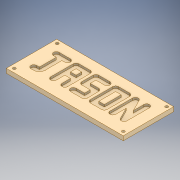
# Autodesk Inventor part: JASON
Saved by Autodesk Inventor 2017 (Build 210142000, 142)
## iProperties
Created: 2016-09-28
Part Number: JASON
Material: Polyethylene, High Density
Document SubType Name: Modeling
Designer: jhaun
Density: 0.952 g/cm^3
Appearance: Smooth - Off-White
Author: jhaun
Autodesk Inventor part; units mm, degrees
ref_plane "YZ Plane" through (0, 0, 0) normal (1, 0, 0) x (0, 1, 0)
ref_plane "XZ Plane" through (0, 0, 0) normal (0, 1, 0) x (-1, 0, 0)
ref_plane "XY Plane" through (0, 0, 0) normal (0, 0, 1) x (1, 0, 0)
sketch "Sketch1" plane through (0, 0, 0) normal (0, 0, 1) x (1, 0, 0)
  arc A0 (0, 6.5) -> (0, -6.5) centre (0, 0) ccw
  line L0 (0, 6.5) -> (26, 6.5)
  line L1 (0, -6.5) -> (6.5, -6.5)
  arc A1 (26, -6.5) -> (26, 6.5) centre (26, 0) ccw
  line L2 (26, -6.5) -> (19.5, -6.5)
  line L3 (6.5, -6.5) -> (6.5, -45.5)
  line L4 (19.5, -6.5) -> (19.5, -45.5)
  line L5 (6.5, -45.5) -> (0, -45.5)
  arc A2 (0, -45.5) -> (0, -58.5) centre (0, -52) ccw
  line L6 (0, -58.5) -> (6.5, -58.5)
  arc A3 (6.5, -58.5) -> (19.5, -45.5) centre (6.5, -45.5) ccw
  line L7 (39, 0) -> (39, -52)
  arc A4 (39, -52) -> (52, -52) centre (45.5, -52) ccw
  line L8 (52, -52) -> (52, -32.5)
  line L9 (52, -32.5) -> (65, -32.5)
  line L10 (52, -6.5) -> (65, -6.5)
  line L11 (65, -6.5) -> (65, -19.5)
  line L12 (65, -19.5) -> (52, -19.5)
  line L13 (52, -19.5) -> (52, -6.5)
  line L14 (45.5, 6.5) -> (71.5, 6.5)
  line L15 (78, 0) -> (78, -52)
  line L16 (65, -32.5) -> (65, -52)
  arc A5 (65, -52) -> (78, -52) centre (71.5, -52) ccw
  arc A6 (45.5, 6.5) -> (39, 0) centre (45.5, 0) ccw
  arc A7 (78, 0) -> (71.5, 6.5) centre (71.5, 0) ccw
  line L17 (84.5, 0) -> (84.5, -26)
  arc A8 (91, 6.5) -> (84.5, 0) centre (91, 0) ccw
  line L18 (91, 6.5) -> (117, 6.5)
  line L19 (91, -32.5) -> (110.5, -32.5)
  arc A9 (84.5, -26) -> (91, -32.5) centre (91, -26) ccw
  line L20 (97.5, -6.5) -> (97.5, -19.5)
  line L21 (97.5, -6.5) -> (117, -6.5)
  arc A10 (117, -6.5) -> (117, 6.5) centre (117, 0) ccw
  line L22 (97.5, -19.5) -> (117, -19.5)
  arc A11 (123.5, -26) -> (117, -19.5) centre (117, -26) ccw
  line L23 (123.5, -26) -> (123.5, -52)
  line L24 (110.5, -32.5) -> (110.5, -45.5)
  line L25 (110.5, -45.5) -> (91, -45.5)
  arc A12 (91, -45.5) -> (91, -58.5) centre (91, -52) ccw
  arc A13 (117, -58.5) -> (123.5, -52) centre (117, -52) ccw
  line L26 (91, -58.5) -> (117, -58.5)
  line L27 (130, 0.001) -> (130, -51.999)
  line L28 (143, -6.499) -> (143, -45.499)
  line L29 (143, -6.499) -> (156, -6.499)
  line L30 (156, -6.499) -> (156, -45.499)
  line L31 (156, -45.499) -> (143, -45.499)
  arc A14 (136.5, 6.501) -> (130, 0.001) centre (136.5, 0.001) ccw
  line L32 (136.5, 6.501) -> (162.5, 6.501)
  line L33 (136.5, -58.499) -> (162.5, -58.499)
  arc A15 (162.5, -58.499) -> (169, -51.999) centre (162.5, -51.999) ccw
  line L34 (169, -51.999) -> (169, 0.001)
  arc A16 (169, 0.001) -> (162.5, 6.501) centre (162.5, 0.001) ccw
  line L35 (175.5, 0) -> (175.5, -52)
  arc A17 (175.524, -51.4421) -> (188.5, -52) centre (182, -52) ccw
  line L36 (214.5, -52.025) -> (214.5, 0.086)
  line L37 (188.5, -52) -> (188.5, -27.5463)
  line L38 (188.5, -27.5463) -> (202.1857, -54.9308)
  line L39 (201.5, 0.086) -> (201.5, -24.4787)
  line L40 (201.5, -24.4787) -> (187.8143, 2.9058)
  arc A18 (214.5, 0.086) -> (201.5, 0.086) centre (208, 0.086) ccw
  arc A19 (130, -51.9852) -> (136.5, -58.499) centre (136.5, -51.999) ccw
  arc A20 (202.1857, -54.9308) -> (214.5, -52.025) centre (208, -52.025) ccw
  arc A21 (187.8143, 2.9058) -> (175.5, 0) centre (182, 0) ccw
  point P0 (0, 0)
  dimension "d2" = 26
  dimension "d3" = 6.5
  dimension "d4" = 13
  dimension "d11" = 13
  dimension "d12" = 6.5
  dimension "d13" = 13
  dimension "d16" = 39
  dimension "d17" = 39
  dimension "d18" = 6.5
  dimension "d19" = 52
  dimension "d20" = 6.5
  dimension "d22" = 13
  dimension "d23" = 19.5
  dimension "d24" = 13
  dimension "d29" = 13
  dimension "d30" = 13
  dimension "d31" = 13
  dimension "d32" = 13
  dimension "d35" = 26
  dimension "d36" = 52
  dimension "d37" = 13
  dimension "d38" = 6.5
  dimension "d39" = 6.5
  dimension "d46" = 19.5
  dimension "d49" = 6.5
  dimension "d50" = 6.5
  dimension "d51" = 90
  dimension "d52" = 6.5
  dimension "d53" = 26
  dimension "d54" = 6.5
  dimension "d55" = 26
  dimension "d56" = 19.5
  dimension "d57" = 39
  dimension "d58" = 13
  dimension "d59" = 13
  dimension "d60" = 19.5
  dimension "d61" = 13
  dimension "d62" = 19.5
  dimension "d63" = 26
  dimension "d64" = 13
  dimension "d65" = 39
  dimension "d66" = 13
  dimension "d67" = 52
  dimension "d68" = 6.5
  dimension "d69" = 39
  dimension "d70" = 13
  dimension "d71" = 39
  dimension "d72" = 13
  dimension "d73" = 13
  dimension "d74" = 6.5
  dimension "d75" = 90
  dimension "d76" = 26
  dimension "d77" = 13
  dimension "d78" = 6.5
  dimension "d79" = 6.5
  dimension "d84" = 13
  dimension "d86" = 26
  dimension "d87" = 13
  dimension "d89" = 52
  dimension "d90" = 13
  dimension "d93" = 6.5
  dimension "d94" = 6.5
  dimension "d95" = 6.5
  dimension "d96" = 6.5
  constraints: 83 end point, 50 point on circle, 22 centre point, 17 horizontal, 17 vertical, 16 tangent, 3 parallel, 3 perpendicular, 1 coincident
  measures "d2" distance of L0.start L0.end
  measures "d3" distance of L1.start L1.end
  measures "d4" distance between parallel lines of L1 L0
  measures "d11" distance between parallel lines of L2 L0
  measures "d12" distance of L2.start L2.end
  measures "d13" distance between parallel lines of L4 L3
  measures "d16" distance of L1.end L3.end
  measures "d17" distance of L2.end L4.end
  measures "d18" distance of L6.start A2.centre
  measures "d19" distance of L7.end L7.start
  measures "d20" distance of L7.end A4.centre
  measures "d22" distance between parallel lines of L7 L8
  measures "d23" distance of L8.start L8.end
  measures "d24" distance of L8.end L9.end
  measures "d29" distance between parallel lines of L7 L13
  measures "d30" distance between parallel lines of L12 L9
  measures "d31" distance of L12.end L10.start
  measures "d32" distance of L11.end L12.end
  measures "d35" distance of L14.start L14.end
  measures "d36" distance of L15.start L15.end
  measures "d37" distance between parallel lines of L15 L11
  measures "d38" distance from line of point (0, 0) L14
  measures "d39" distance from line of point (0, 0) L0
  measures "d46" distance between parallel lines of L7 L4
  measures "d49" distance from line of point (0, 0) L3
  measures "d50" distance between parallel lines of L15 L17
  measures "d52" distance of L17.start A8.centre
  measures "d53" distance of L18.start L18.end
  measures "d54" distance from line of point (0, 0) L18
  measures "d55" distance of L17.start L17.end
  measures "d56" distance of L19.start L19.end
  measures "d57" distance between parallel lines of L19 L18
  measures "d58" distance of L20.start L20.end
  measures "d59" distance between parallel lines of L20 L17
  measures "d60" distance of L20.start L21.end
  measures "d61" distance between parallel lines of L18 L21
  measures "d62" distance of L20.end L22.end
  measures "d63" distance of L23.start L23.end
  measures "d64" distance of L19.end L24.end
  measures "d65" distance between parallel lines of L23 L17
  measures "d66" distance between parallel lines of L23 L24
  measures "d67" distance of L27.start L27.end
  measures "d68" distance between parallel lines of L23 L27
  measures "d69" distance of L28.start L28.end
  measures "d70" distance between parallel lines of L27 L28
  measures "d71" distance of L29.end L30.end
  measures "d72" distance of L28.start L29.end
  measures "d73" distance of L30.end L28.end
  measures "d74" distance of A14.end A14.centre
  measures "d76" distance of L32.start L32.end
  measures "d77" distance between parallel lines of L29 L32
  measures "d78" distance between parallel lines of L35 L34
  measures "d79" distance of A17.start A17.centre
  measures "d84" distance between parallel lines of L35 L37
  measures "d86" distance between parallel lines of L39 L35
  measures "d87" distance between parallel lines of L36 L39
  measures "d89" distance of L35.start L35.end
  measures "d90" distance between parallel lines of L40 L38
  measures "d93" distance of L33.start A19.centre
  measures "d94" distance of L35.start A21.centre
  measures "d95" distance of L36.start A20.centre
  measures "d96" distance of L34.end A16.centre
sketch "Sketch2" plane through (0, 0, 0) normal (0, 0, 1) x (1, 0, 0)
  circle A0 centre (231.3583, -77.1833) radius 3.175
  circle A1 centre (-20, 22) radius 3.175
  circle A2 centre (232, 22) radius 3.175
  circle A3 centre (-19.6417, -77.1833) radius 3.175
  line L0 (-29, 30) -> (240, 30)
  line L1 (240, 30) -> (240, -86)
  line L2 (240, -86) -> (-29, -86)
  line L3 (-29, -86) -> (-29, 30)
  point P0 (0, 0)
  dimension "d99" = 6.35
  dimension "d100" = 6.35
  dimension "d101" = 6.35
  dimension "d102" = 6.35
  dimension "d107" = 269
  dimension "d108" = 116
  constraints: 8 end point, 4 centre point, 2 parallel, 1 horizontal, 1 perpendicular
  measures "d99" diameter of A0
  measures "d100" diameter of A1
  measures "d101" diameter of A2
  measures "d102" diameter of A3
  measures "d107" distance of L0.start L0.end
  measures "d108" distance of L0.end L1.end
extrude "Extrusion1" add sketch "Sketch2" against normal blind 10
extrude "Extrusion2" cut sketch "Sketch1" against normal blind 5
body "Solid1"
